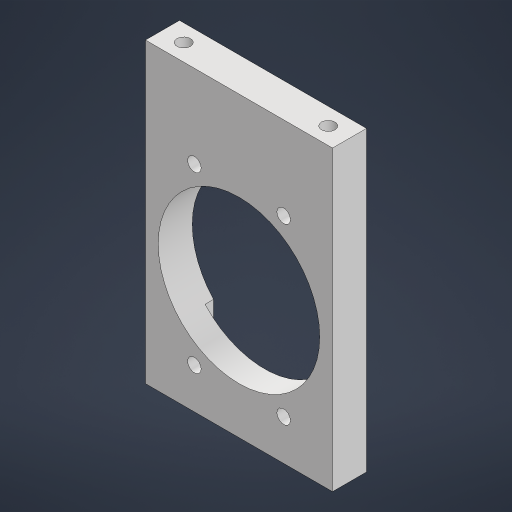
# Autodesk Inventor part: MotorMount_main
Saved by Autodesk Inventor 2024.2 (Build 282272000, 272)
## iProperties
Created: 2023-12-20
Part Number: MotorMount_main
Material: 一般
Document SubType Name: Modeling
Designer: Hanaoka
Density: 1 g/cm^3
Appearance: 既定
Author: Hanaoka
Autodesk Inventor part; units mm, degrees
ref_plane "YZ Plane" through (0, 0, 0) normal (1, 0, 0) x (0, 1, 0)
ref_plane "XZ Plane" through (0, 0, 0) normal (0, 1, 0) x (-1, 0, 0)
ref_plane "XY Plane" through (0, 0, 0) normal (0, 0, 1) x (1, 0, 0)
sketch "スケッチ1" plane through (0, 0, 0) normal (0, 0, 1) x (1, 0, 0)
  line L0 (-11, 20) -> (11, 20)
  line L1 (11, 20) -> (11, -15)
  line L2 (11, -15) -> (-11, -15)
  line L3 (-11, -15) -> (-11, 20)
  line L4 (0, -22) -> (0, 27) projected
  circle A0 centre (0, 0) radius 9.5
  point P0 (0, 20)
  dimension "d0" = 22
  dimension "d1" = 20
  dimension "d2" = 15
  dimension "d3" = 19
  constraints: 8 end point, 2 parallel, 1 centre point, 1 coincident, 1 horizontal, 1 midpoint, 1 perpendicular, 1 point on line
  measures "d0" distance of L0.start L0.end
  measures "d1" vertical distance of point (0, 0) L0.end
  measures "d2" vertical distance of L1.end point (0, 0)
  measures "d3" diameter of A0
extrude "押し出し1" add sketch "スケッチ1" along normal blind 4 contours L0 L4 A0 L2 L3 | L0 L1 L2 L4 A0
derived "MotorMount_sub.ipt"
sketch "スケッチ1_1" plane through (0, 0, 0) normal (0, 0, 1) x (1, 0, 0)
  circle A0 centre (0, 0) radius 2.5
  circle A1 centre (0, 0) radius 6
  circle A2 centre (0, 0) radius 9.5
  circle A3 centre (0, 7.5) radius 1
  circle A4 centre (0, 0) radius 7.5 construction
  line L0 (0, -20.3) -> (0, 20.3)
  circle A5 centre (-6.4952, -3.75) radius 1
  circle A6 centre (6.4952, -3.75) radius 1
  circle A7 centre (0, 0) radius 14.5 construction
  line L1 (-7, 6.4226) -> (-7, 10.9226)
  line L2 (-6, 11.9226) -> (6, 11.9226)
  line L3 (7, 10.9226) -> (7, 6.4226)
  arc A8 (-6, 11.9226) -> (-7, 10.9226) centre (-6, 10.9226) ccw
  arc A9 (7, 10.9226) -> (6, 11.9226) centre (6, 10.9226) ccw
  circle A10 centre (5.25, 10.2317) radius 2 construction
  circle A11 centre (5.25, 10.2317) radius 0.8
  circle A12 centre (-5.25, 10.2317) radius 2 construction
  circle A13 centre (-5.25, 10.2317) radius 0.8
  line L4 (-5.25, 10.2317) -> (-5.25, 7.9175) construction
  line L5 (5.25, 10.2317) -> (5.25, 7.9175) construction
  circle A14 centre (5.25, -10.2317) radius 0.8
  line L6 (7, -6.4226) -> (7, -10.9226)
  arc A15 (6, -11.9226) -> (7, -10.9226) centre (6, -10.9226) ccw
  line L7 (6, -11.9226) -> (-6, -11.9226)
  circle A16 centre (-5.25, -10.2317) radius 2 construction
  line L8 (-7, -10.9226) -> (-7, -6.4226)
  arc A17 (-7, -10.9226) -> (-6, -11.9226) centre (-6, -10.9226) ccw
  circle A18 centre (-5.25, -10.2317) radius 0.8
  circle A19 centre (5.25, -10.2317) radius 2 construction
extrude "押し出し2" cut sketch "スケッチ1_1" along normal blind 1 contours L0 L7 A17 L8 A2 | A2 L6 A15 L7 L0 | L0 L2 A9 L3 A2 | A2 L1 A8 L2 L0
extrude "押し出し3" cut sketch "スケッチ1_1" along normal up to surface (4 mm away) contours A11 | A13 | A14 | A18
sketch "スケッチ3" plane through (-11, 20, 0) normal (0, 1, 0) x (1, 0, 0)
  circle A0 centre (2.5, -2) radius 0.8
  circle A1 centre (19.5, -2) radius 0.8
  line L0 (2.5, -2) -> (0, -2)
  line L1 (0, 0) -> (0, -4) projected
  line L2 (19.5, -2) -> (22, -2)
  line L3 (22, 0) -> (22, -4) projected
  point P0 (11, 0)
  dimension "d12" = 1.6
  dimension "d13" = 2.5
  constraints: 4 end point, 2 centre point, 2 midpoint, 1 collinear, 1 equal radius, 1 horizontal, 1 horizontal alignment, 1 point on line
  measures "d12" diameter of A0
  measures "d13" distance of L0.start L0.end
extrude "押し出し4" cut sketch "スケッチ3" against normal blind 5
sketch "スケッチ4" plane through (-11, -15, 0) normal (0, -1, 0) x (1, 0, 0)
  circle A0 centre (19.5, 2) radius 0.8 projected
  circle A1 centre (2.5, 2) radius 0.8 projected
  line L0 (22, 0) -> (0, 0) projected
  line L1 (0, 0) -> (0, 4) projected
  line L2 (22, 4) -> (0, 4) projected
  line L3 (22, 0) -> (22, 4) projected
  point P0 (11, 0)
extrude "押し出し5" cut sketch "スケッチ4" against normal blind 5 contours A0 | A1
